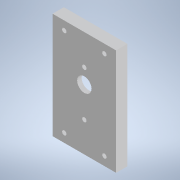
# Autodesk Inventor part: converter_case
Saved by Autodesk Inventor 2021 (Build 250183000, 183)
## iProperties
Created: 2021-01-09
Part Number: converter_case
Material: Generic
Document SubType Name: Modeling
Designer: Mateusz
Density: 1 g/cm^3
Appearance: Default
Author: Mateusz
Autodesk Inventor part; units mm, degrees
ref_plane "YZ Plane" through (0, 0, 0) normal (1, 0, 0) x (0, 1, 0)
ref_plane "XZ Plane" through (0, 0, 0) normal (0, 1, 0) x (-1, 0, 0)
ref_plane "XY Plane" through (0, 0, 0) normal (0, 0, 1) x (1, 0, 0)
sketch "Sketch1" plane through (0, 0, 0) normal (0, 0, 1) x (1, 0, 0)
  line L0 (-1.75, -53.75) -> (-1.75, 11.25) projected
  line L1 (35.25, -53.75) -> (-1.75, -53.75) projected
  line L2 (35.25, 11.25) -> (35.25, -53.75) projected
  line L3 (-1.75, 11.25) -> (35.25, 11.25) projected
  circle A0 centre (30, 8) radius 3 projected
  circle A1 centre (3.5, -50.5) radius 3 projected
  circle A2 centre (30, -50.5) radius 3 projected
  circle A3 centre (3.5, 8) radius 3 projected
  circle A4 centre (3.5, -50.5) radius 1.45
  circle A5 centre (30, -50.5) radius 1.45
  circle A6 centre (30, 8) radius 1.45
  circle A7 centre (3.5, 8) radius 1.45
  point P0 (0, 0)
  dimension "d0" = 2.9
  dimension "d1" = 2.9
  dimension "d2" = 2.9
  dimension "d3" = 2.9
  constraints: 4 centre point
  measures "d0" diameter of A4
  measures "d1" diameter of A5
  measures "d2" diameter of A6
  measures "d3" diameter of A7
extrude "Extrusion1" add sketch "Sketch1" along normal blind 3 contours L0 L3 L2 L1 | A0 | A1 | A2 | A3
sketch "Sketch2" plane through (0, 0, 0) normal (0, 0, -1) x (-1, 0, 0)
  line L0 (-35.25, -53.75) -> (-35.25, 11.25) projected
  line L1 (-35.25, 11.25) -> (-35.75, 11.25)
  line L2 (-35.75, 11.25) -> (-37.75, 11.25)
  line L3 (-37.75, 11.25) -> (-37.75, 11.75)
  line L4 (-37.75, 11.75) -> (-37.75, 13.75)
  line L5 (-37.75, 13.75) -> (1.75, 13.75)
  line L6 (1.75, 13.75) -> (2.25, 13.75)
  line L7 (2.25, 13.75) -> (4.25, 13.75)
  line L8 (4.25, 13.75) -> (4.25, -53.75)
  line L9 (4.25, -53.75) -> (4.25, -54.25)
  line L10 (4.25, -54.25) -> (4.25, -56.25)
  line L11 (4.25, -56.25) -> (-35.25, -56.25)
  line L12 (-35.25, -56.25) -> (-37.75, -56.25)
  line L13 (-37.75, -56.25) -> (-37.75, 11.25)
  line L14 (-37.75, 11.75) -> (4.25, 11.75)
  line L15 (1.75, 11.25) -> (1.75, -53.75) projected
  line L16 (1.75, 11.25) -> (1.75, 11.75)
  line L17 (2.25, 13.75) -> (2.25, -56.25)
  line L18 (1.75, -53.75) -> (4.25, -53.75)
  line L19 (4.25, -54.25) -> (-35.25, -54.25)
  line L20 (1.75, -53.75) -> (-35.25, -53.75) projected
  line L21 (-35.25, -54.25) -> (-37.75, -54.25)
  line L22 (-35.25, -53.75) -> (-35.25, -54.25)
  line L23 (-35.75, 11.25) -> (-35.75, -56.25)
  line L24 (-35.25, 11.25) -> (1.75, 11.25) projected
  line L25 (-35.75, 11.25) -> (-35.75, 13.75)
  point P0 (0, 0)
  point P1 (-35.75, -54.25)
  point P2 (-35.75, 11.75)
  point P3 (2.25, 11.75)
  point P4 (2.25, -54.25)
  dimension "d6" = 0.5
  dimension "d7" = 2
  dimension "d8" = 0.5
  dimension "d9" = 2
  dimension "d10" = 0.5
  dimension "d11" = 2
  dimension "d12" = 0.5
  dimension "d13" = 2
  constraints: 44 end point, 15 point on line, 12 perpendicular, 1 horizontal, 1 parallel
  measures "d6" distance of L0.end L1.end
  measures "d7" distance of L1.end L2.end
  measures "d8" distance of L2.end L3.end
  measures "d9" distance of L3.end L4.end
  measures "d10" distance of L5.end L6.end
  measures "d11" distance of L6.end L7.end
  measures "d12" distance of L8.end L9.end
  measures "d13" distance of L9.end L10.end
extrude "Extrusion2" add sketch "Sketch2" against normal up to surface (3 mm away) contours L22 L21 L23 L1 L0 | L20 L18 L17 L19 L22 | L1 L25 L14 L16 L24 | L15 L16 L14 L17 L18 | L19 L17 L11 L12 L23 L21 | L23 L21 L13 L2 | L2 L3 L14 L25 | L18 L9 L19 L17 | L17 L14 L8 L18 | L19 L10 L11 L17 | L23 L12 L13 L21 | L25 L5 L6 L17 L14 | L14 L4 L5 L25 | L17 L7 L8 L14
extrude "Extrusion3" add sketch "Sketch1" against normal blind 3 contours A0 | A1 | A2 | A3
extrude "Extrusion4" add sketch "Sketch2" along normal blind 4.5 contours L19 L17 L11 L12 L23 L21 | L23 L21 L13 L2 | L2 L3 L14 L25 | L18 L9 L19 L17 | L17 L14 L8 L18 | L19 L10 L11 L17 | L23 L12 L13 L21 | L25 L5 L6 L17 L14 | L14 L4 L5 L25 | L17 L7 L8 L14
sketch "Sketch3" plane through (0, 0, 0) normal (0, 0, -1) x (-1, 0, 0)
  line L0 (-35.75, 11.75) -> (2.25, 11.75) projected
  line L1 (-16.75, 11.75) -> (-16.75, -54.25)
  line L2 (2.25, -54.25) -> (-35.75, -54.25) projected
  circle A0 centre (-16.75, -6.3689) radius 1.45
  circle A1 centre (-16.75, -6.3689) radius 3
  line L3 (-16.75, -6.3689) -> (-16.75, -36.3689)
  circle A2 centre (-16.75, -36.3689) radius 1.45
  circle A3 centre (-16.75, -36.3689) radius 3
  point P0 (0, 0)
  dimension "d20" = 2.9
  dimension "d21" = 6
  dimension "d22" = 30
  dimension "d23" = 2.9
  dimension "d24" = 6
  constraints: 4 centre point, 4 end point, 3 coincident, 2 midpoint, 2 point on line
  measures "d20" diameter of A0
  measures "d21" diameter of A1
  measures "d22" distance of L3.start L3.end
  measures "d23" diameter of A2
  measures "d24" diameter of A3
extrude "Extrusion5" cut sketch "Sketch3" against normal up to surface (3 mm away) contours A0 L1 | L1 A0 | A2 L1 | L1 A2
extrude "Extrusion6" cut sketch "Sketch3" against normal blind 1 contours A1 L1 A0 | L1 A0 A1 | A3 L1 A2 | L1 A2 A3
sketch "Sketch4" plane through (0, 0, 0) normal (0, 0, -1) x (-1, 0, 0)
  circle A0 centre (-16.75, -16.3009) radius 4.767
  point P0 (0, 0)
  point P1 (-16.75, -6.3689)
  dimension "d30" = 9.534
  constraints: 1 centre point
  measures "d30" diameter of A0
extrude "Extrusion7" cut sketch "Sketch4" against normal up to surface (3 mm away)
equation "\"d14\" = d7"
body "Solid1"
